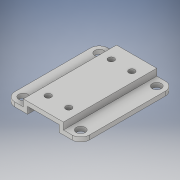
# Autodesk Inventor part: buckconverter-holder
Saved by Autodesk Inventor 2018 (Build 220112000, 112)
## iProperties
Created: 2019-05-07
Part Number: buckconverter-holder
Material: Generic
Document SubType Name: Modeling
Designer: jklei
Density: 1 g/cm^3
Appearance: Default
Author: jklei
Autodesk Inventor part; units mm, degrees
ref_plane "YZ Plane" through (0, 0, 0) normal (1, 0, 0) x (0, 1, 0)
ref_plane "XZ Plane" through (0, 0, 0) normal (0, 1, 0) x (-1, 0, 0)
ref_plane "XY Plane" through (0, 0, 0) normal (0, 0, 1) x (1, 0, 0)
sketch "Sketch1" plane through (0, 0, 0) normal (0, 0, 1) x (1, 0, 0)
  line L0 (0, 0) -> (10, 0)
  line L1 (10, 0) -> (10, 3.175)
  line L2 (10, 3.175) -> (24.605, 3.175)
  line L3 (24.605, 3.175) -> (24.605, 0)
  line L4 (24.605, 0) -> (34.605, 0)
  line L5 (0, 2) -> (8, 2)
  line L6 (8, 2) -> (8, 5.175)
  line L7 (8, 5.175) -> (26.605, 5.175)
  line L8 (26.605, 5.175) -> (26.605, 2)
  line L9 (26.605, 2) -> (34.605, 2)
  line L10 (0, 2) -> (0, 0)
  line L11 (34.605, 0) -> (34.605, 2)
  dimension "d0" = 10
  dimension "d1" = 3.175
  dimension "d2" = 14.605
  dimension "d3" = 10
  dimension "d4" = 2
  constraints: 24 end point, 6 perpendicular, 2 point on line, 1 horizontal, 1 parallel, 1 vertical, 4 other
  measures "d0" distance of L0.start L0.end
  measures "d1" distance of L0.end L1.end
  measures "d2" distance of L1.end L2.end
  measures "d3" distance of L3.end L4.end
  measures "d4" distance between parallel lines of L2 L7
extrude "Extrusion1" add sketch "Sketch1" along normal blind 43.18
sketch "Sketch2" plane through (10, 3.175, 0) normal (0, -1, 0) x (1, 0, 0)
  line L0 (0, 0) -> (14.605, 0) projected
  line L1 (14.605, 0) -> (14.605, 43.18) projected
  line L2 (0, 43.18) -> (14.605, 43.18) projected
  line L3 (0, 0) -> (0, 43.18) projected
  line L4 (14.605, 0) -> (14.605, 43.18) projected
  line L5 (14.605, 0) -> (14.605, 6.985)
  line L6 (14.605, 6.985) -> (12.065, 6.985)
  circle A0 centre (12.065, 6.985) radius 1.3891
  line L7 (0, 0) -> (14.605, 0) projected
  line L8 (0, 0) -> (0, 6.985)
  line L9 (0, 0) -> (0, 43.18) projected
  line L10 (0, 6.985) -> (2.54, 6.985)
  circle A1 centre (2.54, 6.985) radius 1.3891
  line L11 (14.605, 43.18) -> (14.605, 36.195)
  line L12 (14.605, 36.195) -> (12.065, 36.195)
  circle A2 centre (12.065, 36.195) radius 1.3891
  line L13 (-10, 43.18) -> (0, 43.18) projected
  line L14 (0, 43.18) -> (0, 36.195)
  line L15 (0, 36.195) -> (2.54, 36.195)
  circle A3 centre (2.54, 36.195) radius 1.3891
  point P0 (-10, 0)
  dimension "d7" = 6.985
  dimension "d8" = 2.54
  dimension "d9" = 2.7781
  dimension "d10" = 6.985
  dimension "d11" = 2.54
  dimension "d12" = 2.7781
  dimension "d13" = 6.985
  dimension "d14" = 2.54
  dimension "d15" = 2.7781
  dimension "d16" = 6.985
  dimension "d17" = 2.54
  dimension "d18" = 2.7781
  constraints: 16 end point, 4 centre point, 4 coincident, 4 perpendicular, 4 point on line
  measures "d7" distance of L0.end L5.end
  measures "d8" distance of L5.end L6.end
  measures "d9" diameter of A0
  measures "d10" distance of L0.start L8.end
  measures "d11" distance of L8.end L10.end
  measures "d12" diameter of A1
  measures "d13" distance of L1.end L11.end
  measures "d14" distance of L11.end L12.end
  measures "d15" diameter of A2
  measures "d16" distance of L2.start L14.end
  measures "d17" distance of L14.end L15.end
  measures "d18" diameter of A3
extrude "Extrusion2" cut sketch "Sketch2" against normal blind 43.18 contours A0 | A1 | A2 | A3
fillet "Fillet1" radius 4 4 edges at (34.605, 1, 43.18) (34.605, 1, 0) (0, 1, 0) (0, 1, 43.18)
sketch "Sketch4" plane through (26.605, 2, 43.18) normal (0, 1, 0) x (1, 0, 0)
  arc A0 (-26.605, 4) -> (-22.605, 0) centre (-22.605, 4) ccw projected
  arc A1 (-22.605, 43.18) -> (-26.605, 39.18) centre (-22.605, 39.18) ccw projected
  arc A2 (8, 39.18) -> (4, 43.18) centre (4, 39.18) ccw projected
  arc A3 (4, 0) -> (8, 4) centre (4, 4) ccw projected
  circle A4 centre (4, 4) radius 2.1
  circle A5 centre (4, 39.18) radius 2.1
  circle A6 centre (-22.605, 39.18) radius 2.1
  circle A7 centre (-22.605, 4) radius 2.1
  point P0 (-26.605, 43.18)
  dimension "d22" = 4.2
  dimension "d23" = 4.2
  dimension "d24" = 4.2
  dimension "d25" = 4.2
  constraints: 4 centre point, 4 coincident
  measures "d22" diameter of A4
  measures "d23" diameter of A5
  measures "d24" diameter of A6
  measures "d25" diameter of A7
extrude "Extrusion3" cut sketch "Sketch4" against normal blind 43.18
body "Solid1"
